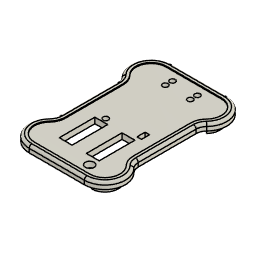
tiny-scarab-v0.2-cover (Autodesk Fusion 360 design; units mm, degrees)
Autodesk Fusion 360 part; units mm, degrees
sketch "drawing" plane through (0, 0, 0) normal (0, 0, 1) x (1, 0, 0)
  circle A0 centre (76.25, -27.495) radius 1.5
  circle A1 centre (114.25, -27.495) radius 1.5
  circle A2 centre (76.25, -87.495) radius 1.5
  circle A3 centre (114.25, -87.495) radius 1.5
  line L0 (79.75, -21.495) -> (110.75, -21.495)
  line L1 (79.75, -93.495) -> (110.75, -93.495)
  line L2 (77.25, -41.2424) -> (77.25, -73.7476)
  line L3 (113.25, -41.2424) -> (113.25, -73.7476)
  arc A4 (79.75, -21.495) -> (74.3929, -34.2439) centre (79.75, -28.995) ccw
  arc A5 (116.1071, -34.2439) -> (110.75, -21.495) centre (110.75, -28.995) ccw
  arc A6 (74.3929, -80.7461) -> (79.75, -93.495) centre (79.75, -85.995) ccw
  arc A7 (110.75, -93.495) -> (116.1071, -80.7461) centre (110.75, -85.995) ccw
  circle A8 centre (76.25, -27.495) radius 3
  circle A9 centre (114.25, -27.495) radius 3
  circle A10 centre (76.25, -87.495) radius 3
  circle A11 centre (114.25, -87.495) radius 3
  line L4 (72.25, -21.495) -> (72.25, -93.495) construction
  line L5 (118.25, -21.495) -> (118.25, -93.495) construction
  circle A12 centre (88.25, -25.495) radius 1.535
  circle A13 centre (88.25, -29.495) radius 1.535
  circle A14 centre (83.25, -26.495) radius 1.5
  circle A15 centre (83.25, -34.995) radius 1.5
  line L6 (95.25, -21.495) -> (95.25, -93.495) construction
  line L7 (90.75, -21.495) -> (99.75, -21.495) construction
  line L8 (99.75, -21.495) -> (99.75, -28.995) construction
  line L9 (99.75, -28.995) -> (90.75, -28.995) construction
  line L10 (90.75, -28.995) -> (90.75, -21.495) construction
  circle A16 centre (106.68, -60.325) radius 0.25 construction
  line L11 (104.93, -55.8) -> (108.43, -55.8) construction
  line L12 (108.43, -55.8) -> (108.43, -64.85) construction
  line L13 (108.43, -64.85) -> (104.93, -64.85) construction
  line L14 (104.93, -64.85) -> (104.93, -55.8) construction
  arc A17 (77.25, -41.2424) -> (74.3929, -34.2439) centre (67.25, -41.2424) ccw
  line L15 (79.75, -28.995) -> (79.75, -21.495) construction
  line L16 (79.75, -28.995) -> (74.3929, -34.2439) construction
  line L17 (67.25, -41.2424) -> (77.25, -41.2424) construction
  line L18 (67.25, -41.2424) -> (74.3929, -34.2439) construction
  arc A18 (116.1071, -34.2439) -> (113.25, -41.2424) centre (123.25, -41.2424) ccw
  arc A19 (74.3929, -80.7461) -> (77.25, -73.7476) centre (67.25, -73.7476) ccw
  arc A20 (113.25, -73.7476) -> (116.1071, -80.7461) centre (123.25, -73.7476) ccw
  circle A21 centre (102.25, -25.495) radius 1.535
  circle A22 centre (102.25, -29.495) radius 1.535
  circle A23 centre (87.75, -62.495) radius 1.535
  line L19 (105.43, -58.075) -> (107.93, -58.075)
  line L20 (107.93, -58.075) -> (107.93, -62.575)
  line L21 (107.93, -62.575) -> (105.43, -62.575)
  line L22 (105.43, -62.575) -> (105.43, -58.075)
  line L23 (105.93, -60.575) -> (107.43, -60.575) construction
  line L24 (107.43, -60.575) -> (107.43, -62.075) construction
  line L25 (107.43, -62.075) -> (105.93, -62.075) construction
  line L26 (105.93, -62.075) -> (105.93, -60.575) construction
  line L27 (105.93, -58.575) -> (107.43, -58.575) construction
  line L28 (107.43, -58.575) -> (107.43, -60.075) construction
  line L29 (107.43, -60.075) -> (105.93, -60.075) construction
  line L30 (105.93, -60.075) -> (105.93, -58.575) construction
  line L31 (106.68, -60.075) -> (106.68, -60.575) construction
  line L32 (81, -24.245) -> (85.5, -24.245) construction
  line L33 (85.5, -24.245) -> (85.5, -28.745) construction
  line L34 (85.5, -28.745) -> (81, -28.745) construction
  line L35 (81, -28.745) -> (81, -24.245) construction
  circle A24 centre (88.25, -25.495) radius 1.9 construction
  circle A25 centre (88.25, -29.495) radius 1.9 construction
  circle A26 centre (102.25, -25.495) radius 1.9 construction
  circle A27 centre (102.25, -29.495) radius 1.9 construction
  circle A28 centre (87.75, -62.495) radius 1.9 construction
  line L36 (81, -32.745) -> (85.5, -32.745) construction
  line L37 (85.5, -32.745) -> (85.5, -37.245) construction
  line L38 (85.5, -37.245) -> (81, -37.245) construction
  line L39 (81, -37.245) -> (81, -32.745) construction
  circle A29 centre (107.25, -26.495) radius 1.5
  line L40 (105, -24.245) -> (109.5, -24.245) construction
  line L41 (109.5, -24.245) -> (109.5, -28.745) construction
  line L42 (109.5, -28.745) -> (105, -28.745) construction
  line L43 (105, -28.745) -> (105, -24.245) construction
  circle A30 centre (105.75, -89.495) radius 1.5
  line L44 (103.5, -87.245) -> (108, -87.245) construction
  line L45 (108, -87.245) -> (108, -91.745) construction
  line L46 (108, -91.745) -> (103.5, -91.745) construction
  line L47 (103.5, -91.745) -> (103.5, -87.245) construction
  line L48 (85.03, -65.882) -> (90.23, -65.882) construction
  line L49 (90.23, -65.882) -> (90.23, -83.882) construction
  line L50 (90.23, -83.882) -> (85.03, -83.882) construction
  line L51 (85.03, -83.882) -> (85.03, -65.882) construction
  line L52 (100.27, -65.882) -> (105.47, -65.882) construction
  line L53 (105.47, -65.882) -> (105.47, -83.882) construction
  line L54 (105.47, -83.882) -> (100.27, -83.882) construction
  line L55 (100.27, -83.882) -> (100.27, -65.882) construction
  line L56 (91.23, -64.882) -> (91.23, -84.882)
  line L57 (91.23, -84.882) -> (84.03, -84.882)
  line L58 (84.03, -84.882) -> (84.03, -64.882)
  line L59 (84.03, -64.882) -> (91.23, -64.882)
  line L60 (106.47, -84.882) -> (99.27, -84.882)
  line L61 (99.27, -84.882) -> (99.27, -64.882)
  line L62 (99.27, -64.882) -> (106.47, -64.882)
  line L63 (106.47, -64.882) -> (106.47, -84.882)
  point P0 (87.63, -74.882)
  point P1 (102.87, -74.882)
  dimension "d1" = 76.25
  dimension "d2" = 3
  dimension "d3" = 27.495
  dimension "d4" = 3
  dimension "d5" = 38
  dimension "d6" = 27.495
  dimension "d7" = 1.5
  dimension "d8" = 3.5
  dimension "d9" = 15
  dimension "d10" = 3.5
  dimension "d11" = 1.5
  dimension "d12" = 15
  dimension "d13" = 60
  dimension "d14" = 3
  dimension "d15" = 76.25
  dimension "d16" = 38
  dimension "d17" = 60
  dimension "d18" = 3
  dimension "d19" = 3.5
  dimension "d20" = 1.5
  dimension "d21" = 3.5
  dimension "d22" = 1.5
  dimension "d23" = 15
  dimension "d24" = 15
  dimension "d31" = 6
  dimension "d32" = 6
  dimension "d33" = 6
  dimension "d34" = 6
  dimension "d35" = 72
  dimension "d36" = 46
  dimension "d37" = 6
  dimension "d38" = 5
  dimension "d39" = 5
  dimension "d40" = 4
  dimension "d41" = 4
  dimension "d42" = 12
  dimension "d43" = 2
  dimension "d44" = 3.07
  dimension "d45" = 4
  dimension "d46" = 3.07
  dimension "d47" = 7
  dimension "d48" = 1
  dimension "d49" = 3
  dimension "d50" = 3
  dimension "d51" = 8.5
  dimension "d52" = 19
  dimension "d53" = 4.5
  dimension "d54" = 4.5
  dimension "d55" = 7.5
  dimension "d56" = 106.68
  dimension "d57" = 60.325
  dimension "d58" = 0.5
  dimension "d59" = 4.525
  dimension "d62" = 1.75
  dimension "d75" = 20
  dimension "d76" = 134.415
  dimension "d77" = 44.415
  dimension "d78" = 20
  dimension "d79" = 20
  dimension "d80" = 20
  dimension "d92" = 3.07
  dimension "d93" = 3.07
  dimension "d94" = 14
  dimension "d95" = 3.07
  dimension "d96" = 33
  dimension "d97" = 0.5
  dimension "d98" = 1.25
  dimension "d100" = 1.5
  dimension "d101" = 0.75
  dimension "d102" = 1.5
  dimension "d103" = 0.75
  dimension "d104" = 3.5
  dimension "d105" = 0.5
  dimension "d106" = 1.5
  dimension "d107" = 3.5
  dimension "d108" = 9.05
  dimension "d109" = 2.25
  dimension "d110" = 2.25
  dimension "d111" = 2.5
  dimension "d112" = 0.5
  dimension "d113" = 0.5
  dimension "d114" = 2.25
  dimension "d115" = 4.5
  dimension "d116" = 4.5
  dimension "d117" = 2.25
  dimension "d118" = 3.8
  dimension "d119" = 3.8
  dimension "d120" = 3.8
  dimension "d121" = 3.8
  dimension "d122" = 3.8
  dimension "d123" = 4.5
  dimension "d124" = 4.5
  dimension "d125" = 2.25
  dimension "d126" = 2.25
  dimension "d127" = 5
  dimension "d128" = 3
  dimension "d129" = 2.25
  dimension "d130" = 2.25
  dimension "d131" = 4.5
  dimension "d132" = 4.5
  dimension "d133" = 105.75
  dimension "d134" = 89.495
  dimension "d135" = 3
  dimension "d136" = 4.5
  dimension "d137" = 4.5
  dimension "d138" = 2.25
  dimension "d139" = 2.25
  dimension "d140" = 4
  dimension "d141" = 12.5
  dimension "d142" = 18
  dimension "d143" = 18
  dimension "d144" = 5.2
  dimension "d145" = 5.2
  dimension "d146" = 102.87
  dimension "d147" = 87.63
  dimension "d148" = 74.882
  dimension "d149" = 2.6
  dimension "d150" = 2.6
  dimension "d151" = 9
  dimension "d152" = 9
  dimension "d153" = -1
  dimension "d154" = -1
  constraint tangent L0 A4
  constraint tangent L0 A5
  constraint tangent L1 A6
  constraint tangent L1 A7
  constraint concentric A0 A8
  constraint concentric A1 A9
  constraint concentric A2 A10
  constraint concentric A3 A11
  constraint vertical L4
  constraint tangent A6 L4
  constraint coincident L0 L4.start
  constraint coincident L1 L4.end
  constraint vertical L5
  constraint coincident L0 L5.start
  constraint coincident L1 L5.end
  constraint tangent A7 L5
  constraint vertical A12.centre A13.centre
  constraint vertical A14.centre A15.centre
  constraint coincident L0 L6.start
  constraint coincident L1 L6.end
  constraint perpendicular L1 L6
  constraint horizontal L7
  constraint vertical L8
  constraint horizontal L9
  constraint vertical L10
  constraint coincident L0 L7.start
  constraint horizontal L11
  constraint vertical L12
  constraint horizontal L13
  constraint vertical L14
  constraint tangent A4 A17
  constraint tangent L2 A17
  constraint coincident A4.centre L15.start
  constraint coincident A17.centre L17.start
  constraint tangent A5 A18
  constraint tangent L3 A18
  constraint tangent A6 A19
  constraint tangent L2 A19
  constraint tangent A7 A20
  constraint tangent L3 A20
  constraint vertical A21.centre A22.centre
  constraint horizontal A12.centre A21.centre
  constraint horizontal A13.centre A22.centre
  constraint horizontal L19
  constraint vertical L20
  constraint horizontal L21
  constraint vertical L22
  constraint horizontal L23
  constraint vertical L24
  constraint horizontal L25
  constraint vertical L26
  constraint horizontal L27
  constraint vertical L28
  constraint horizontal L29
  constraint vertical L30
  constraint midpoint L29 L31.start
  constraint midpoint L23 L31.end
  constraint midpoint A16.centre L31
  constraint horizontal L32
  constraint vertical L33
  constraint horizontal L34
  constraint vertical L35
  constraint concentric A12 A24
  constraint concentric A13 A25
  constraint concentric A21 A26
  constraint concentric A22 A27
  constraint concentric A23 A28
  constraint horizontal L36
  constraint vertical L37
  constraint horizontal L38
  constraint vertical L39
  constraint horizontal A14.centre A29.centre
  constraint horizontal L40
  constraint vertical L41
  constraint horizontal L42
  constraint vertical L43
  constraint horizontal L44
  constraint vertical L45
  constraint horizontal L46
  constraint vertical L47
  constraint horizontal L48
  constraint vertical L49
  constraint horizontal L50
  constraint vertical L51
  constraint horizontal L52
  constraint vertical L53
  constraint horizontal L54
  constraint vertical L55
  constraint horizontal P0 P1
  measures "d1" horizontal distance of origin A0.centre
  measures "d2" diameter of A0
  measures "d3" vertical distance of origin A0.centre
  measures "d4" diameter of A1
  measures "d5" horizontal distance of A0.centre A1.centre
  measures "d6" vertical distance of origin A1.centre
  measures "d7" vertical distance of A0.centre A4.centre
  measures "d8" horizontal distance of A0.centre A4.centre
  measures "d9" diameter of A4
  measures "d10" horizontal distance of A1.centre A5.centre
  measures "d11" vertical distance of A1.centre A5.centre
  measures "d12" diameter of A5
  measures "d13" vertical distance of A0.centre A2.centre
  measures "d14" diameter of A2
  measures "d15" horizontal distance of origin A2.centre
  measures "d16" horizontal distance of A2.centre A3.centre
  measures "d17" distance of A1.centre A3.centre
  measures "d18" diameter of A3
  measures "d19" horizontal distance of A3.centre A7.centre
  measures "d20" vertical distance of A3.centre A7.centre
  measures "d21" horizontal distance of A2.centre A6.centre
  measures "d22" vertical distance of A2.centre A6.centre
  measures "d23" diameter of A6
  measures "d24" diameter of A7
  measures "d31" diameter of A8
  measures "d32" diameter of A9
  measures "d33" diameter of A10
  measures "d34" diameter of A11
  measures "d35" distance of L0 L1
  measures "d36" distance of L4 L5
  measures "d37" distance of A1.centre L0
  measures "d38" distance of L3 L5
  measures "d39" distance of L2 L4
  measures "d40" distance of A2.centre L4
  measures "d41" distance of A3.centre L5
  measures "d42" horizontal distance of A0.centre A12.centre
  measures "d43" vertical distance of A0.centre A12.centre
  measures "d44" diameter of A12
  measures "d45" vertical distance of A12.centre A13.centre
  measures "d46" diameter of A13
  measures "d47" horizontal distance of A0.centre A14.centre
  measures "d48" vertical distance of A0.centre A14.centre
  measures "d49" diameter of A14
  measures "d50" diameter of A15
  measures "d51" distance of A14.centre A15.centre
  measures "d52" distance of A2.centre L6
  measures "d53" distance of L6 L8
  measures "d54" distance of L6 L10
  measures "d55" distance of L0 L9
  measures "d56" horizontal distance of origin A16.centre
  measures "d57" vertical distance of origin A16.centre
  measures "d58" diameter of A16
  measures "d59" distance of A16.centre L11
  measures "d62" distance of A16.centre L12
  measures "d75" diameter of A17
  measures "d76" angle of L15 L16
  measures "d77" angle of L17 L18
  measures "d78" diameter of A18
  measures "d79" diameter of A19
  measures "d80" diameter of A20
  measures "d92" diameter of A21
  measures "d93" diameter of A22
  measures "d94" horizontal distance of A12.centre A21.centre
  measures "d95" diameter of A23
  measures "d96" vertical distance of A13.centre A23.centre
  measures "d97" horizontal distance of A13.centre A23.centre
  measures "d98" distance of A16.centre L20
  measures "d100" distance of L24 L26
  measures "d101" distance of A16.centre L24
  measures "d102" distance of L28 L30
  measures "d103" distance of A16.centre L28
  measures "d104" distance of L25 L27
  measures "d105" distance of L23 L29
  measures "d106" distance of L23 L25
  measures "d107" distance of L12 L14
  measures "d108" distance of L11 L13
  measures "d109" distance of A16.centre L19
  measures "d110" distance of A16.centre L21
  measures "d111" distance of L20 L22
  measures "d112" distance of L22 L30
  measures "d113" distance of L21 L25
  measures "d114" distance of A14.centre L32
  measures "d115" distance of L32 L34
  measures "d116" distance of L33 L35
  measures "d117" distance of A14.centre L35
  measures "d118" diameter of A24
  measures "d119" diameter of A25
  measures "d120" diameter of A26
  measures "d121" diameter of A27
  measures "d122" diameter of A28
  measures "d123" distance of L37 L39
  measures "d124" distance of L36 L38
  measures "d125" distance of A15.centre L37
  measures "d126" distance of A15.centre L38
  measures "d127" horizontal distance of A21.centre A29.centre
  measures "d128" diameter of A29
  measures "d129" distance of A29.centre L40
  measures "d130" distance of A29.centre L41
  measures "d131" distance of L40 L42
  measures "d132" distance of L41 L43
  measures "d133" horizontal distance of origin A30.centre
  measures "d134" vertical distance of origin A30.centre
  measures "d135" diameter of A30
  measures "d136" distance of L45 L47
  measures "d137" distance of L44 L46
  measures "d138" distance of A30.centre L44
  measures "d139" distance of A30.centre L45
  measures "d140" distance of L1 A30.centre
  measures "d141" distance of L5 A30.centre
  measures "d142" distance of L52 L54
  measures "d143" distance of L48 L50
  measures "d144" distance of L49 L51
  measures "d145" distance of L53 L55
  measures "d146" horizontal distance of origin P1
  measures "d147" horizontal distance of origin P0
  measures "d148" vertical distance of origin P0
  measures "d149" distance of L53 P1
  measures "d150" distance of L49 P0
  measures "d151" distance of L52 P1
  measures "d152" distance of L48 P0
sketch "board_cutout" plane through (0, 0, 0) normal (0, 0, 1) x (1, 0, 0)
  circle A0 centre (76.25, -27.495) radius 1.5
  circle A1 centre (114.25, -27.495) radius 1.5
  circle A2 centre (76.25, -87.495) radius 1.5
  circle A3 centre (114.25, -87.495) radius 1.5
  line L0 (79.75, -21.495) -> (110.75, -21.495)
  arc A4 (79.75, -21.495) -> (74.3929, -34.2439) centre (79.75, -28.995) ccw
  arc A5 (77.25, -41.2424) -> (74.3929, -34.2439) centre (67.25, -41.2424) ccw
  line L1 (77.25, -41.2424) -> (77.25, -73.7476)
  arc A6 (74.3929, -80.7461) -> (77.25, -73.7476) centre (67.25, -73.7476) ccw
  arc A7 (74.3929, -80.7461) -> (79.75, -93.495) centre (79.75, -85.995) ccw
  line L2 (79.75, -93.495) -> (110.75, -93.495)
  arc A8 (110.75, -93.495) -> (116.1071, -80.7461) centre (110.75, -85.995) ccw
  arc A9 (113.25, -73.7476) -> (116.1071, -80.7461) centre (123.25, -73.7476) ccw
  line L3 (113.25, -41.2424) -> (113.25, -73.7476)
  arc A10 (116.1071, -34.2439) -> (113.25, -41.2424) centre (123.25, -41.2424) ccw
  arc A11 (116.1071, -34.2439) -> (110.75, -21.495) centre (110.75, -28.995) ccw
  dimension "d182" = 72
  measures "d182" distance of L0 L2
sketch "board_cutout_4mm_offset" plane through (0, 0, 0) normal (0, 0, 1) x (1, 0, 0)
  line L0 (79.75, -21.495) -> (110.75, -21.495) construction
  arc A0 (79.75, -21.495) -> (74.3929, -34.2439) centre (79.75, -28.995) ccw construction
  arc A1 (77.25, -41.2424) -> (74.3929, -34.2439) centre (67.25, -41.2424) ccw construction
  line L1 (77.25, -41.2424) -> (77.25, -73.7476) construction
  arc A2 (74.3929, -80.7461) -> (77.25, -73.7476) centre (67.25, -73.7476) ccw construction
  arc A3 (74.3929, -80.7461) -> (79.75, -93.495) centre (79.75, -85.995) ccw construction
  line L2 (79.75, -93.495) -> (110.75, -93.495) construction
  arc A4 (110.75, -93.495) -> (116.1071, -80.7461) centre (110.75, -85.995) ccw construction
  arc A5 (113.25, -73.7476) -> (116.1071, -80.7461) centre (123.25, -73.7476) ccw construction
  line L3 (113.25, -41.2424) -> (113.25, -73.7476) construction
  arc A6 (116.1071, -34.2439) -> (113.25, -41.2424) centre (123.25, -41.2424) ccw construction
  arc A7 (116.1071, -34.2439) -> (110.75, -21.495) centre (110.75, -28.995) ccw construction
  arc A8 (117.25, -73.7476) -> (118.9643, -77.9467) centre (123.25, -73.7476) ccw
  arc A9 (110.75, -97.495) -> (118.9643, -77.9467) centre (110.75, -85.995) ccw
  line L4 (79.75, -97.495) -> (110.75, -97.495)
  arc A10 (71.5357, -77.9467) -> (79.75, -97.495) centre (79.75, -85.995) ccw
  arc A11 (71.5357, -77.9467) -> (73.25, -73.7476) centre (67.25, -73.7476) ccw
  line L5 (73.25, -41.2424) -> (73.25, -73.7476)
  arc A12 (73.25, -41.2424) -> (71.5357, -37.0433) centre (67.25, -41.2424) ccw
  arc A13 (79.75, -17.495) -> (71.5357, -37.0433) centre (79.75, -28.995) ccw
  line L6 (79.75, -17.495) -> (110.75, -17.495)
  arc A14 (118.9643, -37.0433) -> (110.75, -17.495) centre (110.75, -28.995) ccw
  arc A15 (118.9643, -37.0433) -> (117.25, -41.2424) centre (123.25, -41.2424) ccw
  line L7 (117.25, -41.2424) -> (117.25, -73.7476)
  dimension "d81" = -4
  dimension "d183" = 80
  measures "d183" distance of L4 L6
sketch "pillars" plane through (0, 0, 0) normal (0, 0, 1) x (1, 0, 0)
  arc A0 (79.75, -21.495) -> (74.3929, -34.2439) centre (79.75, -28.995) ccw
  arc A1 (77.25, -41.2424) -> (74.3929, -34.2439) centre (67.25, -41.2424) ccw construction
  line L0 (77.25, -41.2424) -> (77.25, -73.7476) construction
  arc A2 (74.3929, -80.7461) -> (77.25, -73.7476) centre (67.25, -73.7476) ccw construction
  arc A3 (74.3929, -80.7461) -> (79.75, -93.495) centre (79.75, -85.995) ccw
  line L1 (79.75, -93.495) -> (110.75, -93.495) construction
  arc A4 (110.75, -93.495) -> (116.1071, -80.7461) centre (110.75, -85.995) ccw
  arc A5 (113.25, -73.7476) -> (116.1071, -80.7461) centre (123.25, -73.7476) ccw construction
  line L2 (113.25, -41.2424) -> (113.25, -73.7476) construction
  arc A6 (116.1071, -34.2439) -> (113.25, -41.2424) centre (123.25, -41.2424) ccw construction
  arc A7 (116.1071, -34.2439) -> (110.75, -21.495) centre (110.75, -28.995) ccw
  line L3 (79.75, -21.495) -> (110.75, -21.495) construction
  circle A8 centre (76.25, -27.495) radius 1.5 construction
  circle A9 centre (114.25, -27.495) radius 1.5 construction
  circle A10 centre (76.25, -27.495) radius 3 construction
  circle A11 centre (114.25, -27.495) radius 3 construction
  circle A12 centre (76.25, -87.495) radius 1.5 construction
  circle A13 centre (76.25, -87.495) radius 3 construction
  circle A14 centre (114.25, -87.495) radius 1.5 construction
  circle A15 centre (114.25, -87.495) radius 3 construction
  spline S0 degree 2 poles (79.75, -21.495) (79.75, -28.995) (74.3929, -34.2439) knots 0 0 0 1.458918 1.458918 1.458918 weights 1 4 1
  spline S1 degree 2 poles (110.75, -21.495) (110.75, -28.995) (116.1071, -34.2439) knots 0 0 0 1.458918 1.458918 1.458918 weights 1 4 1
  spline S2 degree 2 poles (74.3929, -80.7461) (79.75, -85.995) (79.75, -93.495) knots 0 0 0 1.458918 1.458918 1.458918 weights 1 4 1
  spline S3 degree 2 poles (110.75, -93.495) (110.75, -85.995) (116.1071, -80.7461) knots 0 0 0 1.458918 1.458918 1.458918 weights 1 4 1
  dimension "d181" = 72
  constraint coincident A0.end A1.end
  constraint coincident A0.start L3.start
  constraint coincident A6.start A7.start
  constraint coincident A7.end L3.end
  constraint coincident A3.end L1.start
  constraint coincident A2.start A3.start
  constraint coincident A4.end A5.end
  constraint coincident L1.end A4.start
  measures "d181" distance of L1 L3
sketch "srew_holes" plane through (0, 0, 0) normal (0, 0, 1) x (1, 0, 0)
  circle A0 centre (76.25, -27.495) radius 1.5
  circle A1 centre (114.25, -27.495) radius 1.5
  circle A2 centre (76.25, -87.495) radius 1.5
  circle A3 centre (114.25, -87.495) radius 1.5
  line L0 (79.75, -21.495) -> (110.75, -21.495)
  line L1 (79.75, -93.495) -> (110.75, -93.495)
  dimension "d178" = 72
  dimension "d179" = 72
  dimension "d180" = 31
  measures "d178" distance of L0 L1
  measures "d179" distance of L0 L1
  measures "d180" distance of L0.start L0.end
extrude "Extrude5" add sketch "pillars" along normal blind 4 makes body 1 at (116.0352, -23.6737, 2.6667) makes body 2 at (118.1619, -87.1412, 2.6667) makes body 3 at (72.9424, -32.1424, 2.6667) makes body 4 at (72.403, -87.5019, 2.6667)
extrude "Extrude6" add sketch "board_cutout_4mm_offset" along normal blind 3.7 from surface at 4 separate body makes body 5
sketch "led_cutouts" plane through (0, 0, 0) normal (0, 0, 1) x (1, 0, 0)
  circle A0 centre (88.25, -25.495) radius 1.535
  circle A1 centre (88.25, -29.495) radius 1.535
  circle A2 centre (102.25, -25.495) radius 1.535
  circle A3 centre (102.25, -29.495) radius 1.535
  circle A4 centre (87.75, -62.495) radius 1.535
sketch "button_cutouts" plane through (0, 0, 0) normal (0, 0, 1) x (1, 0, 0)
  circle A0 centre (83.25, -26.495) radius 1.5 construction
  circle A1 centre (83.25, -34.995) radius 1.5 construction
  circle A2 centre (107.25, -26.495) radius 1.5 construction
  circle A3 centre (105.75, -89.495) radius 1.5 construction
  line L0 (105.43, -58.075) -> (107.93, -58.075)
  line L1 (105.43, -62.575) -> (105.43, -58.075)
  line L2 (107.93, -62.575) -> (105.43, -62.575)
  line L3 (107.93, -58.075) -> (107.93, -62.575)
  circle A4 centre (105.75, -89.495) radius 2.5
  dimension "d185" = 3
  dimension "d186" = 1
  dimension "d187" = 5
  measures "d185" diameter of A3
  measures "d187" diameter of A4
sketch "pinheader_cutouts" plane through (0, 0, 0) normal (0, 0, 1) x (1, 0, 0)
  line L0 (91.23, -84.882) -> (84.03, -84.882)
  line L1 (84.03, -84.882) -> (84.03, -64.882)
  line L2 (84.03, -64.882) -> (91.23, -64.882)
  line L3 (91.23, -64.882) -> (91.23, -84.882)
  line L4 (99.27, -64.882) -> (106.47, -64.882)
  line L5 (99.27, -84.882) -> (99.27, -64.882)
  line L6 (106.47, -84.882) -> (99.27, -84.882)
  line L7 (106.47, -64.882) -> (106.47, -84.882)
extrude "Extrude8" cut sketch "led_cutouts" along normal through all bodies 5
extrude "Extrude9" cut sketch "button_cutouts" along normal through all bodies 5
extrude "Extrude10" cut sketch "pinheader_cutouts" along normal through all bodies 5
sketch "screw_sinkholes" plane through (0, 0, 0) normal (0, 0, 1) x (1, 0, 0)
  circle A0 centre (76.25, -27.495) radius 1.5 construction
  circle A1 centre (114.25, -27.495) radius 1.5 construction
  circle A2 centre (76.25, -87.495) radius 1.5 construction
  circle A3 centre (114.25, -87.495) radius 1.5 construction
  circle A4 centre (76.25, -27.495) radius 3
  circle A5 centre (114.25, -27.495) radius 3
  circle A6 centre (76.25, -87.495) radius 3
  circle A7 centre (114.25, -87.495) radius 3
  dimension "d158" = 3
  dimension "d159" = 3
  dimension "d160" = 3
  dimension "d161" = 3
  dimension "d162" = 6
  dimension "d163" = 6
  dimension "d164" = 6
  dimension "d165" = 6
  constraint concentric A0 A4
  constraint concentric A1 A5
  constraint concentric A2 A6
  constraint concentric A3 A7
  measures "d158" diameter of A2
  measures "d159" diameter of A3
  measures "d160" diameter of A0
  measures "d161" diameter of A1
  measures "d162" diameter of A4
  measures "d163" diameter of A5
  measures "d164" diameter of A6
  measures "d165" diameter of A7
sketch "usb_cutout" plane through (0, -17.495, 0) normal (0, 1, 0) x (-1, 0, 0)
  line L0 (-110.75, 4) -> (-79.75, 4)
  line L1 (-79.75, 4) -> (-79.75, 7.7)
  line L2 (-79.75, 7.7) -> (-110.75, 7.7)
  line L3 (-110.75, 7.7) -> (-110.75, 4)
  line L4 (-100.67, 4.58) -> (-89.83, 4.58)
  line L5 (-89.25, 4) -> (-101.25, 4)
  arc A0 (-100.67, 4.58) -> (-101.25, 4) centre (-100.67, 4) ccw
  arc A1 (-89.25, 4) -> (-89.83, 4.58) centre (-89.83, 4) ccw
  dimension "d170" = 0.58
  dimension "d171" = 0.58
  dimension "d172" = 0.58
  dimension "d175" = 12
  constraint horizontal L4
  constraint horizontal L5
  constraint coincident L0 L5.start
  constraint midpoint L0 L5
  constraint tangent L4 A0
  constraint coincident L5.end A0.end
  constraint tangent L4 A1
  constraint coincident L5.start A1.start
  measures "d170" distance of L4 L5
  measures "d171" radius of A0
  measures "d172" radius of A1
  measures "d175" distance of L5.start L5.end
extrude "Extrude12" cut sketch "usb_cutout" against normal blind 4 contours L0 L4 L5 A0 A1 bodies 5
sketch "screw_holes_2.26mm" plane through (0, 0, 0) normal (0, 0, 1) x (1, 0, 0)
  circle A0 centre (76.25, -87.495) radius 1.5 construction
  circle A1 centre (114.25, -87.495) radius 1.5 construction
  circle A2 centre (114.25, -27.495) radius 1.5 construction
  circle A3 centre (76.25, -27.495) radius 1.5 construction
  circle A4 centre (76.25, -27.495) radius 1.13
  circle A5 centre (114.25, -27.495) radius 1.13
  circle A6 centre (76.25, -87.495) radius 1.13
  circle A7 centre (114.25, -87.495) radius 1.13
  dimension "d188" = 2.26
  dimension "d189" = 2.26
  dimension "d190" = 2.26
  dimension "d191" = 2.26
  constraint concentric A3 A4
  constraint concentric A2 A5
  constraint concentric A0 A6
  constraint concentric A1 A7
  measures "d188" diameter of A4
  measures "d189" diameter of A5
  measures "d190" diameter of A6
  measures "d191" diameter of A7
extrude "Extrude13" cut sketch "screw_holes_2.26mm" along normal blind 5 bodies 1 2 3 4 5
sketch "membrane_area" plane through (0, 0, 0) normal (0, 0, 1) x (1, 0, 0)
  arc A0 (79.75, -17.495) -> (71.5357, -37.0433) centre (79.75, -28.995) ccw construction
  line L0 (79.75, -17.495) -> (110.75, -17.495) construction
  arc A1 (118.9643, -37.0433) -> (110.75, -17.495) centre (110.75, -28.995) ccw construction
  arc A2 (118.9643, -37.0433) -> (117.25, -41.2424) centre (123.25, -41.2424) ccw construction
  line L1 (117.25, -41.2424) -> (117.25, -73.7476) construction
  arc A3 (117.25, -73.7476) -> (118.9643, -77.9467) centre (123.25, -73.7476) ccw construction
  arc A4 (110.75, -97.495) -> (118.9643, -77.9467) centre (110.75, -85.995) ccw construction
  line L2 (79.75, -97.495) -> (110.75, -97.495) construction
  arc A5 (71.5357, -77.9467) -> (79.75, -97.495) centre (79.75, -85.995) ccw construction
  arc A6 (71.5357, -77.9467) -> (73.25, -73.7476) centre (67.25, -73.7476) ccw construction
  line L3 (73.25, -41.2424) -> (73.25, -73.7476) construction
  arc A7 (73.25, -41.2424) -> (71.5357, -37.0433) centre (67.25, -41.2424) ccw construction
  arc A8 (114.25, -73.7476) -> (116.8214, -80.0462) centre (123.25, -73.7476) ccw
  arc A9 (110.75, -94.495) -> (116.8214, -80.0462) centre (110.75, -85.995) ccw
  line L4 (79.75, -94.495) -> (110.75, -94.495)
  arc A10 (73.6786, -80.0462) -> (79.75, -94.495) centre (79.75, -85.995) ccw
  arc A11 (73.6786, -80.0462) -> (76.25, -73.7476) centre (67.25, -73.7476) ccw
  line L5 (76.25, -41.2424) -> (76.25, -73.7476)
  arc A12 (76.25, -41.2424) -> (73.6786, -34.9438) centre (67.25, -41.2424) ccw
  arc A13 (79.75, -20.495) -> (73.6786, -34.9438) centre (79.75, -28.995) ccw
  line L6 (79.75, -20.495) -> (110.75, -20.495)
  arc A14 (116.8214, -34.9438) -> (110.75, -20.495) centre (110.75, -28.995) ccw
  arc A15 (116.8214, -34.9438) -> (114.25, -41.2424) centre (123.25, -41.2424) ccw
  line L7 (114.25, -41.2424) -> (114.25, -73.7476)
  dimension "d194" = 3
extrude "Extrude14" cut sketch "membrane_area" against normal blind 0.5 from surface at 7.7 bodies 5
fillet "Fillet1" radius 1.5 12 edges at (69.148, -90.45, 7.7) (95.25, -97.495, 7.7) (121.352, -90.45, 7.7) (117.6951, -76.0153, 7.7) (117.25, -57.495, 7.7) (117.6951, -38.9747, 7.7) (121.352, -24.54, 7.7) (95.25, -17.495, 7.7) (69.148, -24.54, 7.7) (72.8049, -38.9747, 7.7) (73.25, -57.495, 7.7) (72.8049, -76.0153, 7.7) on bodies 5
named bodies: "pillar_tr", "pillar_br", "pillar_tl", "pillar_bl", "cover"
